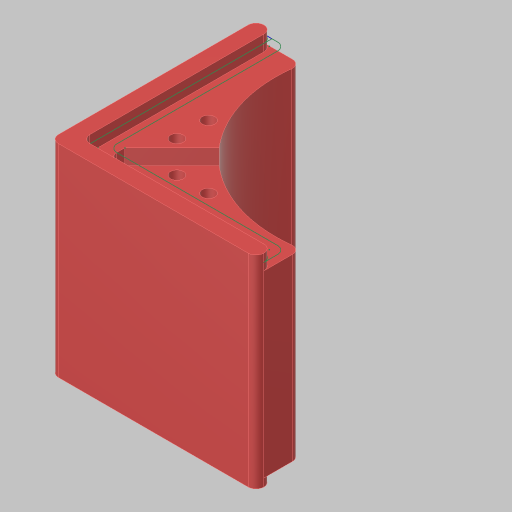
# Autodesk Inventor part: DB1-017
Saved by Autodesk Inventor 2023.5 (Build 275446000, 446)
## iProperties
Created: 2025-03-06
Part Number: DB1-017
Material: PC/ABS Plastic
Document SubType Name: Modeling
Designer: slick
Density: 0.357273 g/cm^3
Appearance: Smooth - Red
Author: slick
Autodesk Inventor part; units mm, degrees
ref_plane "YZ Plane" through (0, 0, 0) normal (1, 0, 0) x (0, 1, 0)
ref_plane "XZ Plane" through (0, 0, 0) normal (0, 1, 0) x (-1, 0, 0)
ref_plane "XY Plane" through (0, 0, 0) normal (0, 0, 1) x (1, 0, 0)
sketch "Sketch1" plane through (0, 0, 0) normal (0, 1, 0) x (-1, 0, 0)
  line L0 (0, 0) -> (-25.4, 0) construction
  line L1 (-25.4, 0) -> (-25.4, -76.2) construction
  line L2 (-25.4, -76.2) -> (0, -76.2) construction
  line L3 (0, -76.2) -> (0, 0) construction
  line L4 (0, 0) -> (-76.2, 0) construction
  line L5 (-76.2, 0) -> (-76.2, -25.4) construction
  line L6 (-76.2, -25.4) -> (0, -25.4) construction
  line L7 (0, -25.4) -> (0, 0) construction
  circle A0 centre (-66.675, -66.675) radius 55.5625 construction
  line L8 (6.35, -82.55) -> (-31.75, -82.55) construction
  line L9 (-31.75, -82.55) -> (-31.75, 6.35) construction
  line L10 (-31.75, 6.35) -> (6.35, 6.35) construction
  line L11 (6.35, 6.35) -> (6.35, -82.55) construction
  line L12 (-82.55, 6.35) -> (6.35, 6.35) construction
  line L13 (6.35, 6.35) -> (6.35, -31.75) construction
  line L14 (6.35, -31.75) -> (-82.55, -31.75) construction
  line L15 (-82.55, -31.75) -> (-82.55, 6.35) construction
  line L16 (-11.935, -76.2) -> (6.35, -76.2)
  line L17 (6.35, -76.2) -> (6.35, 6.35)
  line L18 (6.35, 6.35) -> (-76.2, 6.35)
  line L19 (-76.2, 6.35) -> (-76.2, -11.935)
  arc A1 (-11.935, -76.2) -> (-76.2, -11.935) centre (-66.675, -66.675) ccw
  point P0 (-12.7, -12.7)
  point P1 (-2.7925, -76.2)
  point P2 (-25.4, -12.7)
  point P3 (-38.1, -12.7)
  point P4 (-12.7, -25.4)
  point P5 (-12.7, -38.1)
  dimension "d0" = 25.4
  dimension "d1" = 25.4
  dimension "d2" = 76.2
  dimension "d3" = 76.2
  dimension "d4" = 111.125
  dimension "d5" = 12.7
  dimension "d6" = 12.7
  dimension "d7" = 53.975
  dimension "d9" = 53.975
  dimension "d10" = 6.35
  dimension "d11" = 6.35
  dimension "d14" = 12.7
  dimension "d21" = 12.7
  constraints: 40 end point, 8 parallel, 6 perpendicular, 4 point on circle, 4 point on line, 3 horizontal, 2 centre point, 1 coincident, 1 midpoint, 1 vertical, 10 other
  measures "d0" distance of L4.end L5.end
  measures "d1" distance of L1.end L2.end
  measures "d2" distance of L0.start L4.end
  measures "d3" distance of L2.end L0.start
  measures "d4" diameter of A0
  measures "d5" distance from line of L4 point (-12.7, -12.7)
  measures "d6" distance from line of point (-12.7, -12.7) L3
  measures "d7" horizontal distance of point (-12.7, -12.7) A0.centre
  measures "d9" horizontal distance of point (-12.7, -12.7) A0.centre
  measures "d10" distance between parallel lines of L2 L8
  measures "d11" distance between parallel lines of L4 L12
  measures "d14" distance of point (-12.7, -12.7) point (-25.4, -12.7)
  measures "d21" distance of point (-12.7, -12.7) point (-12.7, -25.4)
extrude "Extrusion1" add sketch "Sketch1" against normal blind 72.0598
hole "Hole1" at (12.7, 0, -12.7) at (25.4, 0, -12.7) at (38.1, 0, -12.7) at (12.7, 0, -25.4) at (12.7, 0, -38.1) direction (0, -1, 0) diameter 5.1054 end through all clearance for "Hex Machine Screw" size "#10" standard "Ansi Unified Screw Threads"
sketch "Sketch2" plane through (0, 0, 0) normal (0, 1, 0) x (1, 0, 0)
  circle A0 centre (12.7, 25.4) radius 2.5527 construction
  circle A1 centre (25.4, 12.7) radius 2.5527 construction
  circle A2 centre (12.7, 12.7) radius 2.5527 construction
  circle A3 centre (38.1, 12.7) radius 2.5527 construction
  circle A4 centre (12.7, 38.1) radius 2.5527 construction
  line L0 (76.2, -6.35) -> (-6.35, -6.35) construction
  line L1 (-6.35, -6.35) -> (-6.35, 76.2) construction
  line L2 (-6.35, 76.2) -> (11.935, 76.2) construction
  arc A5 (11.935, 76.2) -> (76.2, 11.935) centre (66.675, 66.675) ccw construction
  line L3 (76.2, 11.935) -> (76.2, -6.35) construction
  circle A6 centre (12.7, 12.7) radius 4.7625 construction
  line L4 (-6.35, 76.2) -> (11.935, 76.2) construction
  line L5 (5.3975, 76.2) -> (5.3975, 5.3975)
  line L6 (5.3975, 5.3975) -> (76.2, 5.3975)
  line L7 (76.2, 11.935) -> (76.2, -6.35) construction
  line L8 (76.2, 5.3975) -> (76.2, -6.35)
  line L9 (-6.35, -6.35) -> (76.2, -6.35) construction
  line L10 (76.2, -6.35) -> (-6.35, -6.35)
  line L11 (-6.35, -6.35) -> (-6.35, 76.2) construction
  line L12 (-6.35, -6.35) -> (-6.35, 76.2)
  line L13 (-6.35, 76.2) -> (5.3975, 76.2)
  circle A7 centre (12.7, 12.7) radius 7.3025 construction
  point P0 (0, 0)
  dimension "d35" = 9.525
  dimension "d36" = 2.54
  constraints: 12 end point, 2 centre point, 2 collinear, 2 horizontal, 2 point on line, 2 tangent, 1 coincident, 1 perpendicular, 1 vertical
  measures "d35" diameter of A6
  measures "d36" radial gap between concentric circles of A6 A7
extrude "Extrusion2" add sketch "Sketch2" along normal blind 3.048
sketch "Sketch3" plane through (0, 3.048, 0) normal (0, 1, 0) x (1, 0, 0)
  line L0 (-6.35, 76.2) -> (-6.35, -6.35) construction
  line L1 (76.2, -6.35) -> (-6.35, -6.35) construction
  line L2 (-6.35, 76.2) -> (-0.0254, 76.2)
  line L3 (-0.0254, 76.2) -> (-0.0254, -6.35)
  line L4 (-0.0254, -6.35) -> (-6.35, -6.35)
  line L5 (-6.35, -6.35) -> (-6.35, 76.2)
  line L6 (76.2, -6.35) -> (-6.35, -6.35)
  line L7 (-6.35, -6.35) -> (-6.35, -0.0254)
  line L8 (-6.35, -0.0254) -> (76.2, -0.0254)
  line L9 (76.2, -0.0254) -> (76.2, -6.35)
  point P0 (0, 0)
  point P1 (-0.0254, -6.35)
  point P2 (-0.0254, -0.0254)
  dimension "d39" = 6.3246
  dimension "d40" = 6.3246
  constraints: 16 end point, 4 parallel, 2 horizontal, 2 perpendicular, 2 point on line
  measures "d39" distance between parallel lines of L1 L8
  measures "d40" distance of L0.start L2.end
extrude "Extrusion3" add sketch "Sketch3" along normal blind 3.1496
sketch "Sketch4" plane through (0, -72.0598, 0) normal (0, -1, 0) x (1, 0, 0)
  circle A0 centre (12.7, -25.4) radius 2.5527 construction
  circle A1 centre (25.4, -12.7) radius 2.5527 construction
  circle A2 centre (12.7, -12.7) radius 2.5527 construction
  circle A3 centre (38.1, -12.7) radius 2.5527 construction
  circle A4 centre (12.7, -38.1) radius 2.5527 construction
  line L0 (-6.35, 6.35) -> (76.2, 6.35) construction
  line L1 (76.2, 6.35) -> (76.2, -11.935) construction
  arc A5 (76.2, -11.935) -> (11.935, -76.2) centre (66.675, -66.675) ccw construction
  line L2 (11.935, -76.2) -> (-6.35, -76.2) construction
  line L3 (-6.35, -76.2) -> (-6.35, 6.35) construction
  line L4 (76.2, -11.935) -> (76.2, 6.35) construction
  line L5 (-6.35, -76.2) -> (-6.35, 6.35) construction
  line L6 (76.2, 6.35) -> (-6.35, 6.35)
  line L7 (-6.35, 6.35) -> (-6.35, 0.0254)
  line L8 (-6.35, 0.0254) -> (76.2, 0.0254)
  line L9 (76.2, 0.0254) -> (76.2, 6.35)
  line L10 (-6.35, 6.35) -> (-0.0254, 6.35)
  line L11 (-0.0254, 6.35) -> (-0.0254, -76.2)
  line L12 (-0.0254, -76.2) -> (-6.35, -76.2)
  line L13 (-6.35, -76.2) -> (-6.35, 6.35)
  point P0 (0, 0)
  point P1 (-0.0254, 0.0254)
  dimension "d43" = 6.3246
  dimension "d44" = 6.3246
  constraints: 16 end point, 4 parallel, 2 horizontal, 2 perpendicular, 2 point on line
  measures "d43" distance between parallel lines of L0 L8
  measures "d44" distance between parallel lines of L3 L11
extrude "Extrusion4" add sketch "Sketch4" along normal blind 3.1496
fillet "Fillet1" radius 3.175 13 edges at (-6.35, -34.5059, 6.35) (-6.35, -34.5059, -76.2) (11.935, -36.0299, -76.2) (-0.0254, -73.6346, 0.0254) (76.2, -73.6346, 0.0254) (76.2, -34.5059, 6.35) (-0.0254, -73.6346, -76.2) (-0.0254, 4.6228, 0.0254) (5.3975, 1.524, -5.3975) (5.3975, 1.524, -76.2) (76.2, 1.524, -5.3975) (76.2, 4.6228, 0.0254) (76.2, -36.0299, -11.935)
sketch "Sketch5" plane through (0, 0, 0) normal (0, 1, 0) x (1, 0, 0)
  arc A0 (76.2, 8.2818) -> (72.6818, 11.4381) centre (73.025, 8.2818) ccw construction
  arc A1 (11.4381, 72.6818) -> (72.6818, 11.4381) centre (66.675, 66.675) ccw construction
  arc A2 (11.4381, 72.6818) -> (8.2818, 76.2) centre (8.2818, 73.025) ccw construction
  line L0 (8.2818, 76.2) -> (2.2225, 76.2) construction
  arc A3 (5.3975, 73.025) -> (2.2225, 76.2) centre (2.2225, 73.025) ccw construction
  line L1 (5.3975, 73.025) -> (5.3975, 8.5725) construction
  arc A4 (5.3975, 8.5725) -> (8.5725, 5.3975) centre (8.5725, 8.5725) ccw construction
  line L2 (8.5725, 5.3975) -> (73.025, 5.3975) construction
  arc A5 (76.2, 2.2225) -> (73.025, 5.3975) centre (73.025, 2.2225) ccw construction
  line L3 (76.2, 2.2225) -> (76.2, 8.2818) construction
  circle A6 centre (12.7, 25.4) radius 2.5527 construction
  circle A7 centre (25.4, 12.7) radius 2.5527 construction
  circle A8 centre (12.7, 12.7) radius 2.5527 construction
  circle A9 centre (38.1, 12.7) radius 2.5527 construction
  circle A10 centre (12.7, 38.1) radius 2.5527 construction
  line L4 (24.3692, 30.6554) -> (5.3975, 11.6837)
  line L5 (30.6554, 24.3692) -> (11.6837, 5.3975)
  circle A11 centre (12.7, 12.7) radius 2.5527 construction
  line L6 (11.7156, 5.4294) -> (5.4294, 11.7156) construction
  circle A12 centre (12.7, 12.7) radius 4.445 construction
  arc A13 (11.4381, 72.6818) -> (72.6818, 11.4381) centre (66.675, 66.675) ccw construction
  arc A14 (24.3692, 30.6554) -> (30.6554, 24.3692) centre (66.675, 66.675) ccw
  arc A15 (5.3975, 8.5725) -> (8.5725, 5.3975) centre (8.5725, 8.5725) ccw construction
  line L7 (5.3975, 8.5725) -> (5.3975, 73.025) construction
  line L8 (73.025, 5.3975) -> (8.5725, 5.3975) construction
  line L9 (5.3975, 73.025) -> (5.3975, 8.5725) construction
  line L10 (5.4294, 11.7156) -> (5.3975, 8.5725)
  line L11 (8.5725, 5.3975) -> (73.025, 5.3975) construction
  line L12 (11.7156, 5.4294) -> (8.5725, 5.3975)
  arc A16 (5.3975, 8.5725) -> (8.5725, 5.3975) centre (8.5725, 8.5725) ccw
  point P0 (0, 0)
  dimension "d48" = 8.89
  constraints: 10 end point, 7 point on circle, 5 point on line, 4 coincident, 3 centre point, 2 tangent, 1 midpoint, 1 parallel, 1 perpendicular
  measures "d48" diameter of A12
extrude "Extrusion5" cut sketch "Sketch5" against normal blind 6.35
sketch "Sketch6" plane through (0, 3.048, 0) normal (0, 1, 0) x (1, 0, 0)
  arc A0 (76.2, 2.2225) -> (73.025, 5.3975) centre (73.025, 2.2225) ccw projected
  line L0 (73.025, 5.3975) -> (8.5725, 5.3975) projected
  arc A1 (5.3975, 8.5725) -> (8.5725, 5.3975) centre (8.5725, 8.5725) ccw projected
  line L1 (5.3975, 8.5725) -> (5.3975, 73.025) projected
  arc A2 (5.3975, 73.025) -> (2.2225, 76.2) centre (2.2225, 73.025) ccw projected
  line L2 (2.2225, 76.2) -> (-0.0254, 76.2) projected
  line L3 (-0.0254, 76.2) -> (-0.0254, 3.1496) projected
  arc A3 (-0.0254, 3.1496) -> (3.1496, -0.0254) centre (3.1496, 3.1496) ccw projected
  line L4 (3.1496, -0.0254) -> (73.0251, -0.0254) projected
  arc A4 (76.2, -3.175) -> (73.0251, -0.0254) centre (73.0251, -3.2004) ccw projected
  line L5 (76.2, -3.175) -> (76.2, 2.2225) projected
  arc A5 (-0.0254, 73.0251) -> (-3.175, 76.2) centre (-3.2004, 73.0251) ccw projected
  arc A6 (-0.0254, 73.0251) -> (-3.175, 76.2) centre (-3.2004, 73.0251) ccw construction
  arc A7 (-0.0254, 73.0251) -> (-3.175, 76.2) centre (-3.2004, 73.0251) ccw construction
  line L6 (-3.175, 76.2) -> (-0.0254, 76.2)
  point P0 (0, 0)
  point P1 (-6.35, 73.025)
  point P2 (-0.0254, 73.0251)
  constraints: 2 end point, 1 perpendicular
extrude "Extrusion6" cut sketch "Sketch6" against normal up to surface (3.048 mm away)
extrude "Extrusion7" cut sketch "Sketch6" along normal up to surface (3.1496 mm away) contours A5 L6 L3
equation "\"d1\" = d0"
equation "\"d3\" = d2"
equation "\"d9\" = d7"
equation "\"d11\" = d10"
equation "\"d40\" = d39"
equation "\"d43\" = d39"
equation "\"d44\" = d43"
equation "\"d45\" = d41"
equation "\"d41\" = 3.1496"
body "Solid1"
